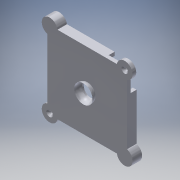
# Autodesk Inventor part: pantalla_case_inferior
Saved by Autodesk Inventor 2019 (Build 230136000, 136)
## iProperties
Created: 2018-11-22
Part Number: pantalla_case_inferior
Material: Steel, Mild, Welded
Document SubType Name: Modeling
Designer: mecanica
Density: 7.85 g/cm^3
Appearance: PTFE
Author: mecanica
Autodesk Inventor part; units mm, degrees
ref_plane "YZ Plane" through (0, 0, 0) normal (1, 0, 0) x (0, 1, 0)
ref_plane "XZ Plane" through (0, 0, 0) normal (0, 1, 0) x (-1, 0, 0)
ref_plane "XY Plane" through (0, 0, 0) normal (0, 0, 1) x (1, 0, 0)
sketch "Sketch1" plane through (0, 0, 0) normal (0, 0, 1) x (1, 0, 0)
  line L0 (-9.4337, -26.8631) -> (-9.4337, 6.6369) projected
  arc A0 (-7.4337, 8.6369) -> (-9.4337, 6.6369) centre (-7.4337, 6.6369) ccw projected
  line L1 (-7.4337, 8.6369) -> (27.5663, 8.6369) projected
  line L2 (27.5663, 11.1369) -> (27.5663, 8.6369) projected
  line L3 (27.5663, 11.1369) -> (-5.0221, 11.1369) projected
  arc A1 (-5.0221, 11.1369) -> (-11.9337, 5.1466) centre (-10.3586, 10.3118) ccw projected
  line L4 (-11.9337, 5.1466) -> (-11.9337, -26.8631) projected
  line L5 (-9.4337, -26.8631) -> (-11.9337, -26.8631) projected
  line L6 (38.0663, -39.3631) -> (8.0663, -39.3631) projected
  line L7 (8.0663, -41.8631) -> (8.0663, -39.3631) projected
  line L8 (8.0663, -41.8631) -> (35.6546, -41.8631) projected
  arc A2 (35.6546, -41.8631) -> (42.5663, -35.8728) centre (40.9912, -41.038) ccw projected
  line L9 (42.5663, -35.8728) -> (42.5663, -3.8631) projected
  line L10 (40.0663, -3.8631) -> (42.5663, -3.8631) projected
  line L11 (40.0663, -3.8631) -> (40.0663, -37.3631) projected
  arc A3 (38.0663, -39.3631) -> (40.0663, -37.3631) centre (38.0663, -37.3631) ccw projected
  point P0 (0, 0)
extrude "Extrusion1" add sketch "Sketch1" along normal blind 4
sketch "Sketch2" plane through (0, 0, 4) normal (0, 0, 1) x (1, 0, 0)
  line L0 (27.5663, 8.6369) -> (38.0663, 8.6369) projected
  arc A0 (40.0663, 6.6369) -> (38.0663, 8.6369) centre (38.0663, 6.6369) ccw projected
  line L1 (40.0663, 6.6369) -> (40.0663, -3.8631) projected
  line L2 (40.0663, -3.8631) -> (42.5663, -3.8631) projected
  line L3 (42.5663, -3.8631) -> (42.5663, 5.1466) projected
  arc A1 (42.5663, 5.1466) -> (35.6546, 11.1369) centre (40.9912, 10.3118) ccw projected
  line L4 (35.6546, 11.1369) -> (27.5663, 11.1369) projected
  line L5 (27.5663, 11.1369) -> (27.5663, 8.6369) projected
  line L6 (-9.4337, -37.3631) -> (-9.4337, -26.8631) projected
  line L7 (-9.4337, -26.8631) -> (-11.9337, -26.8631) projected
  line L8 (-11.9337, -26.8631) -> (-11.9337, -35.8728) projected
  arc A2 (-11.9337, -35.8728) -> (-5.0221, -41.8631) centre (-10.3586, -41.038) ccw projected
  line L9 (-5.0221, -41.8631) -> (8.0663, -41.8631) projected
  line L10 (8.0663, -41.8631) -> (8.0663, -39.3631) projected
  line L11 (8.0663, -39.3631) -> (-7.4337, -39.3631) projected
  arc A3 (-9.4337, -37.3631) -> (-7.4337, -39.3631) centre (-7.4337, -37.3631) ccw projected
  line L12 (-9.4337, -26.8631) -> (-9.4337, 6.6369) projected
  arc A4 (-7.4337, 8.6369) -> (-9.4337, 6.6369) centre (-7.4337, 6.6369) ccw projected
  line L13 (-7.4337, 8.6369) -> (27.5663, 8.6369) projected
  line L14 (27.5663, 8.6369) -> (27.5663, 11.1369) projected
  line L15 (27.5663, 11.1369) -> (-5.0221, 11.1369) projected
  arc A5 (-5.0221, 11.1369) -> (-11.9337, 5.1466) centre (-10.3586, 10.3118) ccw projected
  line L16 (-11.9337, 5.1466) -> (-11.9337, -26.8631) projected
  line L17 (-11.9337, -26.8631) -> (-9.4337, -26.8631) projected
  line L18 (38.0663, -39.3631) -> (8.0663, -39.3631) projected
  line L19 (8.0663, -39.3631) -> (8.0663, -41.8631) projected
  line L20 (8.0663, -41.8631) -> (35.6546, -41.8631) projected
  arc A6 (35.6546, -41.8631) -> (42.5663, -35.8728) centre (40.9912, -41.038) ccw projected
  line L21 (42.5663, -35.8728) -> (42.5663, -3.8631) projected
  line L22 (42.5663, -3.8631) -> (40.0663, -3.8631) projected
  line L23 (40.0663, -3.8631) -> (40.0663, -37.3631) projected
  arc A7 (38.0663, -39.3631) -> (40.0663, -37.3631) centre (38.0663, -37.3631) ccw projected
  point P0 (0, 0)
extrude "Extrusion2" add sketch "Sketch2" along normal blind 2.5 contours L5 L4 A1 L3 L2 L1 A0 L0 | L13 A4 L12 L7 L16 A5 L15 L5 | L2 L21 A6 L20 L10 L18 A7 L23 | L6 A3 L11 L10 L9 A2 L8 L7
sketch "Sketch3" plane through (0, 0, 6.5) normal (0, 0, 1) x (1, 0, 0)
  arc A0 (-7.4337, 8.6369) -> (-9.4337, 6.6369) centre (-7.4337, 6.6369) ccw projected
  line L0 (-9.4337, 6.6369) -> (-9.4337, -37.3631) projected
  arc A1 (-9.4337, -37.3631) -> (-7.4337, -39.3631) centre (-7.4337, -37.3631) ccw projected
  line L1 (-7.4337, -39.3631) -> (38.0663, -39.3631) projected
  arc A2 (38.0663, -39.3631) -> (40.0663, -37.3631) centre (38.0663, -37.3631) ccw projected
  line L2 (40.0663, -37.3631) -> (40.0663, 6.6369) projected
  arc A3 (40.0663, 6.6369) -> (38.0663, 8.6369) centre (38.0663, 6.6369) ccw projected
  line L3 (38.0663, 8.6369) -> (-7.4337, 8.6369) projected
  arc A4 (-2.6837, 5.6369) -> (-2.6837, -0.8631) centre (-2.6837, 2.3869) ccw projected
  line L4 (33.3163, 5.6369) -> (-2.6837, 5.6369) projected
  arc A5 (33.3163, -0.8631) -> (33.3163, 5.6369) centre (33.3163, 2.3869) ccw projected
  line L5 (31.3163, -0.8631) -> (33.3163, -0.8631) projected
  line L6 (31.3163, -29.8631) -> (31.3163, -0.8631) projected
  line L7 (33.3163, -29.8631) -> (31.3163, -29.8631) projected
  arc A6 (33.3163, -36.3631) -> (33.3163, -29.8631) centre (33.3163, -33.1131) ccw projected
  line L8 (-2.6837, -36.3631) -> (33.3163, -36.3631) projected
  arc A7 (-2.6837, -29.8631) -> (-2.6837, -36.3631) centre (-2.6837, -33.1131) ccw projected
  line L9 (-0.6837, -29.8631) -> (-2.6837, -29.8631) projected
  line L10 (-0.6837, -0.8631) -> (-0.6837, -29.8631) projected
  line L11 (-2.6837, -0.8631) -> (-0.6837, -0.8631) projected
  point P0 (0, 0)
extrude "Extrusion3" add sketch "Sketch3" against normal blind 2.5 contours L3 A3 L2 A2 L1 A1 L0 A0 | L4 A5 L5 L6 L7 A6 L8 A7 L9 L10 L11 A4
sketch "Sketch4" plane through (0, 0, 6.5) normal (0, 0, 1) x (1, 0, 0)
  circle A0 centre (15.3163, -15.3631) radius 7.5
  line L0 (42.5663, -35.8728) -> (42.5663, 5.1466) projected
  line L1 (-5.0221, -41.8631) -> (35.6546, -41.8631) projected
  point P0 (0, 0)
  point P1 (42.5663, -15.3631)
  point P2 (15.3163, -41.8631)
  dimension "d6" = 15
  constraints: 2 midpoint, 1 centre point, 1 horizontal alignment, 1 vertical alignment
  measures "d6" diameter of A0
extrude "Extrusion4" add sketch "Sketch4" along normal blind 8.509
sketch "Sketch6" plane through (0, 0, 4) normal (0, 0, -1) x (-1, 0, 0)
  arc A0 (-33.3163, -29.8631) -> (-33.3163, -36.3631) centre (-33.3163, -33.1131) ccw projected
  arc A1 (-33.3163, 5.6369) -> (-33.3163, -0.8631) centre (-33.3163, 2.3869) ccw projected
  arc A2 (2.6837, -0.8631) -> (2.6837, 5.6369) centre (2.6837, 2.3869) ccw projected
  arc A3 (2.6837, -36.3631) -> (2.6837, -29.8631) centre (2.6837, -33.1131) ccw projected
  circle A4 centre (-33.3163, -33.1131) radius 3.25
  circle A5 centre (-33.3163, 2.3869) radius 3.25
  circle A6 centre (2.6837, 2.3869) radius 3.25
  circle A7 centre (2.6837, -33.1131) radius 3.25
  point P0 (0, 0)
  constraints: 4 centre point, 4 coincident, 4 concentric
extrude "Extrusion6" add sketch "Sketch6" along normal blind 3.93
sketch "Sketch7" plane through (0, 0, 0) normal (0, 0, -1) x (-1, 0, 0)
  arc A0 (-42.5663, -35.8728) -> (-35.6546, -41.8631) centre (-40.9912, -41.038) ccw projected
  arc A1 (11.9337, 5.1466) -> (5.0221, 11.1369) centre (10.3586, 10.3118) ccw projected
  circle A2 centre (-40.9912, -41.038) radius 1.8
  circle A3 centre (10.3586, 10.3118) radius 1.8
  point P0 (0, 0)
  dimension "d13" = 3.6
  dimension "d14" = 3.6
  constraints: 2 centre point, 2 coincident
  measures "d13" diameter of A2
  measures "d14" diameter of A3
extrude "Extrusion7" cut sketch "Sketch7" against normal blind 4
sketch "Sketch8" plane through (0, 0, 6.5) normal (0, 0, 1) x (1, 0, 0)
  point P0 (40.9912, 10.3118)
  point P1 (-10.3586, -41.038)
hole "Hole1" at (40.9912, 10.3118, 6.5) at (-10.3586, -41.038, 6.5) direction (0, 0, -1) diameter 2.4 depth 2.5 countersink diameter 4.4 countersink angle 90
body "Solid1"
